LGR Foundation (Autodesk Fusion 360 design; units mm, degrees)
Autodesk Fusion 360 part; units mm, degrees
sketch "Sketch1" plane through (0, 0, 0) normal (0, 0, 1) x (1, 0, 0)
  line L0 (-40, 37.5) -> (40, 37.5)
  line L1 (40, 37.5) -> (40, -37.5)
  line L2 (40, -37.5) -> (-40, -37.5)
  line L3 (-40, -37.5) -> (-40, 37.5)
  dimension "d1" = 80
  dimension "d2" = 75
  dimension "d3" = 37.5
  dimension "d4" = 40
  constraint horizontal L0
  constraint vertical L1
  constraint horizontal L2
  constraint vertical L3
  measures "d1" distance of L1 L3
  measures "d2" distance of L0 L2
  measures "d3" distance of origin L2
  measures "d4" distance of origin L1
extrude "Extrude1" add sketch "Sketch1" along normal blind 6
sketch "Sketch2" plane through (0, 0, 6) normal (0, 0, 1) x (-1, 0, 0)
  line L0 (40, 37.5) -> (-40, 37.5)
  line L1 (-40, 37.5) -> (-40, -37.5)
  line L2 (-40, -37.5) -> (40, -37.5)
  line L3 (40, -37.5) -> (40, 37.5)
  line L4 (26.55, -37.5) -> (22.55, -37.5)
  line L5 (22.55, -37.5) -> (22.55, 37.5)
  line L6 (22.55, 37.5) -> (26.55, 37.5)
  line L7 (26.55, 37.5) -> (26.55, -37.5)
  line L8 (-22.55, -37.5) -> (-26.55, -37.5)
  line L9 (-26.55, -37.5) -> (-26.55, 37.5)
  line L10 (-26.55, 37.5) -> (-22.55, 37.5)
  line L11 (-22.55, 37.5) -> (-22.55, -37.5)
  dimension "d7" = 45.1
  dimension "d8" = 53.1
  dimension "d9" = 13.45
  dimension "d10" = 17.45
  constraint horizontal L4
  constraint vertical L5
  constraint horizontal L6
  constraint vertical L7
  constraint coincident L0 L5.end
  constraint coincident L2 L4.start
  constraint horizontal L8
  constraint vertical L9
  constraint horizontal L10
  constraint vertical L11
  constraint coincident L0 L9.end
  constraint coincident L2 L8.start
  measures "d7" distance of L5 L11
  measures "d8" distance of L7 L9
  measures "d9" distance of L3 L7
  measures "d10" distance of L3 L5
extrude "Extrude2" add sketch "Sketch2" along normal blind 20 contours L0 L2 L4 L5 L6 L7 | L0 L2 L8 L9 L10 L11
sketch "Sketch3" plane through (26.55, 0, 0) normal (1, 0, 0) x (0, 1, 0)
  line L0 (-37.5, 6) -> (37.5, 6)
  line L1 (37.5, 6) -> (37.5, 26)
  line L2 (37.5, 26) -> (-37.5, 26)
  line L3 (-37.5, 26) -> (-37.5, 6)
  circle A0 centre (-18, 20) radius 2.55
  circle A1 centre (18, 20) radius 2.55
  line L4 (37.5, 0) -> (-37.5, 0)
  dimension "d13" = 5.1
  dimension "d14" = 5.1
  dimension "d15" = 20
  dimension "d16" = 36
  dimension "d17" = 19.5
  constraint horizontal A0.centre A1.centre
  measures "d13" diameter of A0
  measures "d14" diameter of A1
  measures "d15" distance of A0.centre L4
  measures "d16" distance of A0.centre A1.centre
  measures "d17" distance of L1 A1.centre
extrude "Extrude3" cut sketch "Sketch3" along normal blind 0 and the other way blind 53.1 contours A0 | A1
chamfer "Chamfer1" distance 2 angle 45 2 edges at (26.55, 0, 6) (-26.55, 0, 6)
sketch "Sketch8" plane through (0, 0, 6) normal (0, 0, 1) x (-1, 0, 0)
  line L0 (28.55, 37.5) -> (28.55, -37.5)
  line L1 (28.55, -37.5) -> (40, -37.5)
  line L2 (40, -37.5) -> (40, 37.5)
  line L3 (40, 37.5) -> (28.55, 37.5)
  line L4 (-40, 37.5) -> (-40, -37.5)
  line L5 (-40, -37.5) -> (-28.55, -37.5)
  point P0 (34, -30)
  point P1 (-34, -30)
  point P2 (-34, 30)
  point P3 (34, 30)
  dimension "d57" = 68
  dimension "d58" = 60
  dimension "d59" = 6
  dimension "d60" = 7.5
  constraint horizontal P0 P1
  constraint vertical P1 P2
  constraint horizontal P2 P3
  constraint vertical P0 P3
  measures "d57" distance of P0 P1
  measures "d58" distance of P1 P2
  measures "d59" distance of P1 L4
  measures "d60" distance of P1 L5
hole "Hole3" at (-34, 30, 6) at (-34, -30, 6) at (34, -30, 6) at (34, 30, 6) direction (0, 0, -1) diameter 3.797 end through all countersink diameter 7.087 countersink angle 100
fillet "Fillet1" radius 5 4 edges at (40, -37.5, 3) (40, 37.5, 3) (-40, -37.5, 3) (-40, 37.5, 3)
fillet "Fillet2" radius 5 4 edges at (24.55, -37.5, 26) (-24.55, -37.5, 26) (-24.55, 37.5, 26) (24.55, 37.5, 26)
sketch "Sketch13" plane through (0, 0, 6) normal (0, 0, 1) x (-1, 0, 0)
  line L0 (-22.55, 37.5) -> (-22.55, -37.5)
  line L1 (-22.55, -37.5) -> (22.55, -37.5)
  line L2 (22.55, -37.5) -> (22.55, 37.5)
  line L3 (22.55, 37.5) -> (-22.55, 37.5)
  line L4 (20.05, 27.1318) -> (20.05, -27.1318)
  line L5 (15.4698, 35) -> (-15.4698, 35)
  line L6 (-20.05, 27.1318) -> (-20.05, -27.1318)
  line L7 (15.4698, -35) -> (-15.4698, -35)
  line L8 (17.234, 27.8516) -> (2.3937, 0.7198)
  line L9 (2.3937, -0.7198) -> (17.234, -27.8516)
  line L10 (16.7858, -32.7802) -> (1.316, -4.4974)
  line L11 (-1.316, -4.4974) -> (-16.7858, -32.7802)
  line L12 (-17.234, -27.8516) -> (-2.3937, -0.7198)
  line L13 (-2.3937, 0.7198) -> (-17.234, 27.8516)
  line L14 (-16.7858, 32.7802) -> (-1.316, 4.4974)
  line L15 (1.316, 4.4974) -> (16.7858, 32.7802)
  arc A0 (20.05, 27.1318) -> (17.234, 27.8516) centre (18.55, 27.1318) ccw
  arc A1 (17.234, -27.8516) -> (20.05, -27.1318) centre (18.55, -27.1318) ccw
  arc A2 (15.4698, -35) -> (16.7858, -32.7802) centre (15.4698, -33.5) ccw
  arc A3 (16.7858, 32.7802) -> (15.4698, 35) centre (15.4698, 33.5) ccw
  arc A4 (-15.4698, 35) -> (-16.7858, 32.7802) centre (-15.4698, 33.5) ccw
  arc A5 (-17.234, 27.8516) -> (-20.05, 27.1318) centre (-18.55, 27.1318) ccw
  arc A6 (-20.05, -27.1318) -> (-17.234, -27.8516) centre (-18.55, -27.1318) ccw
  arc A7 (-16.7858, -32.7802) -> (-15.4698, -35) centre (-15.4698, -33.5) ccw
  arc A8 (1.316, -4.4974) -> (-1.316, -4.4974) centre (0, -5.2172) ccw
  arc A9 (2.3937, 0.7198) -> (2.3937, -0.7198) centre (3.7097, 0) ccw
  arc A10 (-1.316, 4.4974) -> (1.316, 4.4974) centre (0, 5.2172) ccw
  arc A11 (-2.3937, -0.7198) -> (-2.3937, 0.7198) centre (-3.7097, 0) ccw
  point P0 (20.05, 33)
  point P1 (20.05, -33)
  point P2 (18, 35)
  point P3 (-18, 35)
  point P4 (-20.05, 33)
  point P5 (-20.05, -33)
  point P6 (18, -35)
  point P7 (-18, -35)
  dimension "d91" = 2.5
  dimension "d92" = 2.5
  dimension "d93" = 66
  dimension "d95" = 66
  dimension "d96" = 2.5
  dimension "d97" = 36
  dimension "d98" = 36
  dimension "d99" = 2.5
  dimension "d100" = 4.55
  dimension "d101" = 4.55
  dimension "d102" = 4.5
  dimension "d103" = 4.5
  dimension "d104" = 1.5
  constraint vertical L4
  constraint horizontal L5
  constraint parallel L0 L6
  constraint horizontal L7
  constraint parallel L9 L10
  constraint parallel L8 L11
  constraint parallel L11 L12
  constraint parallel L13 L14
  constraint coincident P0 L4
  constraint coincident P0 L8
  constraint tangent L4 A0
  constraint tangent L8 A0
  constraint coincident P1 L4
  constraint coincident P1 L9
  constraint tangent L4 A1
  constraint tangent L9 A1
  constraint equal A0 A1
  constraint coincident P6 L10
  constraint coincident P6 L7
  constraint tangent L10 A2
  constraint tangent L7 A2
  constraint equal A0 A2
  constraint coincident P2 L15
  constraint coincident P2 L5
  constraint tangent L15 A3
  constraint tangent L5 A3
  constraint equal A0 A3
  constraint coincident P3 L14
  constraint coincident P3 L5
  constraint tangent L14 A4
  constraint tangent L5 A4
  constraint equal A0 A4
  constraint coincident P4 L13
  constraint coincident P4 L6
  constraint tangent L13 A5
  constraint tangent L6 A5
  constraint equal A0 A5
  constraint coincident P5 L6
  constraint coincident P5 L12
  constraint tangent L6 A6
  constraint tangent L12 A6
  constraint equal A0 A6
  constraint coincident P7 L11
  constraint coincident P7 L7
  constraint tangent L11 A7
  constraint tangent L7 A7
  constraint equal A0 A7
  constraint tangent L10 A8
  constraint tangent L11 A8
  constraint equal A0 A8
  constraint tangent L9 A9
  constraint tangent L8 A9
  constraint equal A0 A9
  constraint tangent L15 A10
  constraint tangent L14 A10
  constraint equal A0 A10
  constraint tangent L13 A11
  constraint tangent L12 A11
  constraint equal A0 A11
  measures "d91" distance of L2 L4
  measures "d92" distance of L3 L5
  measures "d93" distance of P0 P1
  measures "d95" distance of P4 P5
  measures "d96" distance of L0 L6
  measures "d97" distance of P6 P7
  measures "d98" distance of P2 P3
  measures "d99" distance of L1 L7
  measures "d100" distance of L2 P6
  measures "d101" distance of L2 P2
  measures "d102" distance of L3 P0
  measures "d103" distance of L3 P4
  measures "d104" radius of A0
extrude "Extrude6" cut sketch "Sketch13" along normal blind 0 and the other way blind 6 contours L4 L8 L9 A0 A1 A9 | L5 L14 L15 A3 A4 A10 | L6 L12 L13 A5 A6 A11 | L7 L10 L11 A2 A7 A8
extrude "Extrude7" cut 1 faces at (29.1614, 9.0439, 0) along direction (0, 0, -1) blind 0 and the other way blind 0.4
ref_plane "WorkPlane3" through (34.275, 0, 1.9) normal (0, 0, 1) x (1, 0, 0)
sketch "Sketch14" plane through (0, 0, 1.9) normal (0, 0, 1) x (1, 0, 0)
  circle A0 centre (34, 30) radius 4.5
  circle A1 centre (-34, 30) radius 4.5
  circle A2 centre (-34, -30) radius 4.5
  circle A3 centre (34, -30) radius 4.5
  line L0 (35, 37.5) -> (28.55, 37.5)
  line L1 (40, -32.5) -> (40, 32.5)
  dimension "d115" = 9
  dimension "d116" = 9
  dimension "d117" = 9
  dimension "d118" = 9
  dimension "d119" = 68
  dimension "d120" = 60
  dimension "d121" = 7.5
  dimension "d122" = 6
  constraint horizontal A0.centre A1.centre
  constraint vertical A0.centre A3.centre
  constraint horizontal A2.centre A3.centre
  constraint vertical A1.centre A2.centre
  measures "d115" diameter of A0
  measures "d116" diameter of A1
  measures "d117" diameter of A2
  measures "d118" diameter of A3
  measures "d119" distance of A0.centre A1.centre
  measures "d120" distance of A0.centre A3.centre
  measures "d121" distance of A0.centre L0
  measures "d122" distance of A0.centre L1
ref_plane "WorkPlane4" through (34.275, 0, 0.4) normal (0, 0, 1) x (1, 0, 0)
sketch "Sketch17" plane through (0, 0, 6) normal (0, 0, 1) x (-1, 0, 0)
  arc A0 (-40, -32.5) -> (-35, -37.5) centre (-35, -32.5) ccw
  line L0 (-35, -37.5) -> (-28.55, -37.5)
  line L1 (-28.55, -37.5) -> (-28.55, 37.5)
  line L2 (-28.55, 37.5) -> (-35, 37.5)
  arc A1 (-35, 37.5) -> (-40, 32.5) centre (-35, 32.5) ccw
  line L3 (-40, 32.5) -> (-40, -32.5)
  line L4 (-33.05, -23) -> (-35.5, -23)
  line L5 (-37.5, -21) -> (-37.5, 21)
  line L6 (-35.5, 23) -> (-33.05, 23)
  line L7 (-31.05, 21) -> (-31.05, -21)
  arc A2 (-33.05, -23) -> (-31.05, -21) centre (-33.05, -21) ccw
  arc A3 (-31.05, 21) -> (-33.05, 23) centre (-33.05, 21) ccw
  arc A4 (-35.5, 23) -> (-37.5, 21) centre (-35.5, 21) ccw
  arc A5 (-37.5, -21) -> (-35.5, -23) centre (-35.5, -21) ccw
  line L8 (35.5, -23) -> (33.05, -23)
  line L9 (31.05, -21) -> (31.05, 21)
  line L10 (33.05, 23) -> (35.5, 23)
  line L11 (37.5, 21) -> (37.5, -21)
  line L12 (28.55, -37.5) -> (28.55, 37.5)
  line L13 (40, -32.5) -> (40, 32.5)
  arc A6 (35.5, -23) -> (37.5, -21) centre (35.5, -21) ccw
  arc A7 (31.05, -21) -> (33.05, -23) centre (33.05, -21) ccw
  arc A8 (33.05, 23) -> (31.05, 21) centre (33.05, 21) ccw
  arc A9 (37.5, 21) -> (35.5, 23) centre (35.5, 21) ccw
  circle A10 centre (-34, 30) radius 3.5435
  circle A11 centre (-34, -30) radius 3.5435
  point P0 (-34, -30)
  point P1 (-34, 30)
  point P2 (34, -30)
  point P3 (34, 30)
  dimension "d134" = 2.5
  dimension "d135" = 2.5
  dimension "d136" = 7
  dimension "d137" = 7
  dimension "d138" = 2
  dimension "d141" = 2.5
  dimension "d142" = 2.5
  dimension "d143" = 7
  dimension "d144" = 7
  dimension "d145" = 2
  constraint horizontal L4
  constraint vertical L5
  constraint horizontal L6
  constraint vertical L7
  constraint tangent L4 A2
  constraint tangent L7 A2
  constraint tangent L6 A3
  constraint tangent L7 A3
  constraint equal A2 A3
  constraint tangent L6 A4
  constraint tangent L5 A4
  constraint equal A2 A4
  constraint tangent L5 A5
  constraint tangent L4 A5
  constraint equal A2 A5
  constraint horizontal L8
  constraint vertical L9
  constraint horizontal L10
  constraint vertical L11
  constraint tangent L8 A6
  constraint tangent L11 A6
  constraint tangent L9 A7
  constraint tangent L8 A7
  constraint equal A6 A7
  constraint tangent L9 A8
  constraint tangent L10 A8
  constraint equal A6 A8
  constraint tangent L10 A9
  constraint tangent L11 A9
  constraint equal A6 A9
  measures "d134" distance of L1 L7
  measures "d135" distance of L3 L5
  measures "d136" distance of L4 P0
  measures "d137" distance of L6 P1
  measures "d138" radius of A2
  measures "d141" distance of L9 L12
  measures "d142" distance of L11 L13
  measures "d143" distance of L8 P2
  measures "d144" distance of L10 P3
  measures "d145" radius of A6
extrude "Extrude10" cut sketch "Sketch17" against normal blind 5.6 contours L4 L5 L6 L7 A2 A3 A4 A5 | L8 L9 L10 L11 A6 A7 A8 A9
extrude "Extrude12" add 1 faces at (-23.7167, 7, 0.4) along direction (0, 0, -1) blind 5
sketch "Sketch18" plane through (0, -37.5, 0) normal (0, -1, 0) x (1, 0, 0)
  line L0 (35, -4.6) -> (35, 6)
  line L1 (35, 6) -> (28.55, 6)
  line L2 (28.55, 6) -> (26.55, 8)
  line L3 (26.55, 8) -> (26.55, 21)
  line L4 (26.55, 21) -> (22.55, 21)
  line L5 (22.55, 21) -> (22.55, 6)
  line L6 (22.55, 6) -> (-22.55, 6)
  line L7 (-22.55, 6) -> (-22.55, 21)
  line L8 (-22.55, 21) -> (-26.55, 21)
  line L9 (-26.55, 21) -> (-26.55, 8)
  line L10 (-26.55, 8) -> (-28.55, 6)
  line L11 (-28.55, 6) -> (-35, 6)
  line L12 (-35, 6) -> (-35, -4.6)
  line L13 (-35, -4.6) -> (35, -4.6)
  line L14 (-14.5, 3.5) -> (14.5, 3.5)
  line L15 (16, 2) -> (16, -0.6)
  line L16 (14.5, -2.1) -> (-14.5, -2.1)
  line L17 (-16, -0.6) -> (-16, 2)
  arc A0 (-14.5, 3.5) -> (-16, 2) centre (-14.5, 2) ccw
  arc A1 (-16, -0.6) -> (-14.5, -2.1) centre (-14.5, -0.6) ccw
  arc A2 (14.5, -2.1) -> (16, -0.6) centre (14.5, -0.6) ccw
  arc A3 (16, 2) -> (14.5, 3.5) centre (14.5, 2) ccw
  dimension "d154" = 32
  dimension "d155" = 2.5
  dimension "d156" = 2.5
  dimension "d157" = 16
  dimension "d158" = 1.5
  constraint horizontal L14
  constraint vertical L15
  constraint horizontal L16
  constraint vertical L17
  constraint tangent L14 A0
  constraint tangent L17 A0
  constraint tangent L17 A1
  constraint tangent L16 A1
  constraint equal A0 A1
  constraint tangent L16 A2
  constraint tangent L15 A2
  constraint equal A0 A2
  constraint tangent L15 A3
  constraint tangent L14 A3
  constraint equal A0 A3
  measures "d154" distance of L15 L17
  measures "d155" distance of L6 L14
  measures "d156" distance of L13 L16
  measures "d157" distance of origin L17
  measures "d158" radius of A0
extrude "Extrude13" cut sketch "Sketch18" against normal blind 4 contours L14 L15 L16 L17 A0 A1 A2 A3
sketch "Sketch19" plane through (0, 37.5, 0) normal (0, 1, 0) x (-1, 0, 0)
  line L0 (35, -4.6) -> (35, 6)
  line L1 (35, 6) -> (28.55, 6)
  line L2 (28.55, 6) -> (26.55, 8)
  line L3 (26.55, 8) -> (26.55, 21)
  line L4 (26.55, 21) -> (22.55, 21)
  line L5 (22.55, 21) -> (22.55, 6)
  line L6 (22.55, 6) -> (-22.55, 6)
  line L7 (-22.55, 6) -> (-22.55, 21)
  line L8 (-22.55, 21) -> (-26.55, 21)
  line L9 (-26.55, 21) -> (-26.55, 8)
  line L10 (-26.55, 8) -> (-28.55, 6)
  line L11 (-28.55, 6) -> (-35, 6)
  line L12 (-35, 6) -> (-35, -4.6)
  line L13 (-35, -4.6) -> (35, -4.6)
  line L14 (-14.5, 3.5) -> (14.5, 3.5)
  line L15 (16, 2) -> (16, -0.6)
  line L16 (14.5, -2.1) -> (-14.5, -2.1)
  line L17 (-16, -0.6) -> (-16, 2)
  arc A0 (-14.5, 3.5) -> (-16, 2) centre (-14.5, 2) ccw
  arc A1 (-16, -0.6) -> (-14.5, -2.1) centre (-14.5, -0.6) ccw
  arc A2 (14.5, -2.1) -> (16, -0.6) centre (14.5, -0.6) ccw
  arc A3 (16, 2) -> (14.5, 3.5) centre (14.5, 2) ccw
  dimension "d161" = 2.5
  dimension "d162" = 2.5
  dimension "d163" = 32
  dimension "d164" = 16
  dimension "d165" = 1.5
  constraint horizontal L14
  constraint vertical L15
  constraint horizontal L16
  constraint vertical L17
  constraint tangent L14 A0
  constraint tangent L17 A0
  constraint tangent L17 A1
  constraint tangent L16 A1
  constraint equal A0 A1
  constraint tangent L16 A2
  constraint tangent L15 A2
  constraint equal A0 A2
  constraint tangent L15 A3
  constraint tangent L14 A3
  constraint equal A0 A3
  measures "d161" distance of L13 L16
  measures "d162" distance of L6 L14
  measures "d163" distance of L15 L17
  measures "d164" distance of origin L17
  measures "d165" radius of A0
extrude "Extrude14" cut sketch "Sketch19" against normal blind 4 contours L14 L15 L16 L17 A0 A1 A2 A3
sketch "Sketch20" plane through (-40, 0, 0) normal (-1, 0, 0) x (0, -1, 0)
  line L0 (32.5, -4.6) -> (32.5, 6)
  line L1 (32.5, 6) -> (-32.5, 6)
  line L2 (-32.5, 6) -> (-32.5, -4.6)
  line L3 (-32.5, -4.6) -> (32.5, -4.6)
  line L4 (-21, 3.5) -> (21, 3.5)
  line L5 (23, 1.5) -> (23, -0.1)
  line L6 (21, -2.1) -> (-21, -2.1)
  line L7 (-23, -0.1) -> (-23, 1.5)
  line L8 (-32.5, 6) -> (32.5, 6)
  arc A0 (-21, 3.5) -> (-23, 1.5) centre (-21, 1.5) ccw
  arc A1 (-23, -0.1) -> (-21, -2.1) centre (-21, -0.1) ccw
  arc A2 (21, -2.1) -> (23, -0.1) centre (21, -0.1) ccw
  arc A3 (23, 1.5) -> (21, 3.5) centre (21, 1.5) ccw
  dimension "d168" = 2.5
  dimension "d169" = 2.5
  dimension "d170" = 46
  dimension "d171" = 23
  dimension "d172" = 2
  constraint horizontal L4
  constraint vertical L5
  constraint horizontal L6
  constraint vertical L7
  constraint tangent L4 A0
  constraint tangent L7 A0
  constraint tangent L7 A1
  constraint tangent L6 A1
  constraint equal A0 A1
  constraint tangent L6 A2
  constraint tangent L5 A2
  constraint equal A0 A2
  constraint tangent L5 A3
  constraint tangent L4 A3
  constraint equal A0 A3
  measures "d168" distance of L4 L8
  measures "d169" distance of L3 L6
  measures "d170" distance of L5 L7
  measures "d171" distance of origin L7
  measures "d172" radius of A0
extrude "Extrude15" cut sketch "Sketch20" against normal blind 22 contours L4 L5 L6 L7 A0 A1 A2 A3
sketch "Sketch21" plane through (40, 0, 0) normal (1, 0, 0) x (0, 1, 0)
  line L0 (32.5, -4.6) -> (32.5, 6)
  line L1 (32.5, 6) -> (-32.5, 6)
  line L2 (-32.5, 6) -> (-32.5, -4.6)
  line L3 (-32.5, -4.6) -> (32.5, -4.6)
  line L4 (-21, 3.5) -> (21, 3.5)
  line L5 (23, 1.5) -> (23, -0.1)
  line L6 (21, -2.1) -> (-21, -2.1)
  line L7 (-23, -0.1) -> (-23, 1.5)
  line L8 (21, 6) -> (-21, 6)
  arc A0 (-21, 3.5) -> (-23, 1.5) centre (-21, 1.5) ccw
  arc A1 (-23, -0.1) -> (-21, -2.1) centre (-21, -0.1) ccw
  arc A2 (21, -2.1) -> (23, -0.1) centre (21, -0.1) ccw
  arc A3 (23, 1.5) -> (21, 3.5) centre (21, 1.5) ccw
  dimension "d175" = 2.5
  dimension "d176" = 2.5
  dimension "d177" = 46
  dimension "d178" = 23
  dimension "d179" = 2
  constraint horizontal L4
  constraint vertical L5
  constraint horizontal L6
  constraint vertical L7
  constraint tangent L4 A0
  constraint tangent L7 A0
  constraint tangent L7 A1
  constraint tangent L6 A1
  constraint equal A0 A1
  constraint tangent L6 A2
  constraint tangent L5 A2
  constraint equal A0 A2
  constraint tangent L5 A3
  constraint tangent L4 A3
  constraint equal A0 A3
  measures "d175" distance of L4 L8
  measures "d176" distance of L3 L6
  measures "d177" distance of L5 L7
  measures "d178" distance of origin L5
  measures "d179" radius of A0
extrude "Extrude16" cut sketch "Sketch21" against normal blind 22 contours L4 L5 L6 L7 A0 A1 A2 A3
sketch "Sketch23" plane through (26.55, 0, 0) normal (1, 0, 0) x (0, 1, 0)
  arc A0 (37.5, 21) -> (32.5, 26) centre (32.5, 21) ccw
  line L0 (32.5, 26) -> (-32.5, 26)
  arc A1 (-32.5, 26) -> (-37.5, 21) centre (-32.5, 21) ccw
  line L1 (-37.5, 21) -> (-37.5, 8)
  line L2 (-37.5, 8) -> (37.5, 8)
  line L3 (37.5, 8) -> (37.5, 21)
  circle A2 centre (-18, 20) radius 2.55
  circle A3 centre (18, 20) radius 2.55
  line L4 (-31, 14.95) -> (31, 14.95)
  line L5 (32.5, 13.45) -> (32.5, 12)
  line L6 (31, 10.5) -> (-31, 10.5)
  line L7 (-32.5, 12) -> (-32.5, 13.45)
  arc A4 (-31, 14.95) -> (-32.5, 13.45) centre (-31, 13.45) ccw
  arc A5 (-32.5, 12) -> (-31, 10.5) centre (-31, 12) ccw
  arc A6 (31, 10.5) -> (32.5, 12) centre (31, 12) ccw
  arc A7 (32.5, 13.45) -> (31, 14.95) centre (31, 13.45) ccw
  dimension "d186" = 2.5
  dimension "d187" = 5
  dimension "d188" = 5
  dimension "d189" = 5.05
  dimension "d190" = 1.5
  constraint horizontal L4
  constraint vertical L5
  constraint horizontal L6
  constraint vertical L7
  constraint tangent L4 A4
  constraint tangent L7 A4
  constraint tangent L7 A5
  constraint tangent L6 A5
  constraint equal A4 A5
  constraint tangent L6 A6
  constraint tangent L5 A6
  constraint equal A4 A6
  constraint tangent L5 A7
  constraint tangent L4 A7
  constraint equal A4 A7
  measures "d186" distance of L2 L6
  measures "d187" distance of L1 L7
  measures "d188" distance of L3 L5
  measures "d189" distance of A2.centre L4
  measures "d190" radius of A4
extrude "Extrude17" cut sketch "Sketch23" against normal blind 55 contours L4 L5 L6 L7 A4 A5 A6 A7
equation "d3 = ( 75 / 2 ) * 1 mm"
equation "d4 = ( 80 / 2 ) * 1 mm"
equation "d9 = ( ( 80 - 53.1 ) / 2 ) * 1 mm"
equation "d10 = ( ( 80 - 45.1 ) / 2 ) * 1 mm"
equation "d17 = ( ( 75 - 36 ) / 2 ) * 1 mm"
equation "d59 = ( ( 80 - 68 ) / 2 ) * 1 mm"
equation "d60 = ( ( 75 - 60 ) / 2 ) * 1 mm"
equation "d100 = ( ( 45.1 - 36 ) / 2 ) * 1 mm"
equation "d101 = ( ( 45.1 - 36 ) / 2 ) * 1 mm"
equation "d102 = ( ( 75 - 66 ) / 2 ) * 1 mm"
equation "d103 = ( ( 75 - 66 ) / 2 ) * 1 mm"
equation "d171 = ( 46 / 2 ) * 1 mm"
equation "d189 = ( ( 5.1 / 2 ) * 1 mm ) + 2.5 mm"
